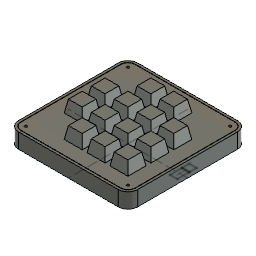
OpenMicro (Autodesk Fusion 360 design; units mm, degrees)
Autodesk Fusion 360 part; units mm, degrees
note: some values were not read from the file. Chosen so that the rebuilt part matches the saved one: which bodies a step acts on.
sketch "Sketch1" plane through (0, 0, 0) normal (0, 1, 0) x (1, 0, 0)
  line L0 (6, 0) -> (89, 0)
  line L1 (95, -6) -> (95, -89)
  line L2 (89, -95) -> (6, -95)
  line L3 (0, -89) -> (0, -6)
  arc A0 (6, 0) -> (0, -6) centre (6, -6) ccw
  arc A1 (95, -6) -> (89, 0) centre (89, -6) ccw
  arc A2 (89, -95) -> (95, -89) centre (89, -89) ccw
  arc A3 (0, -89) -> (6, -95) centre (6, -89) ccw
  line L4 (47.5, 0) -> (47.5, -95) construction
  line L5 (0, -47.5) -> (95, -47.5) construction
  circle A4 centre (5, -5) radius 1
  circle A5 centre (90, -5) radius 1
  circle A6 centre (90, -90) radius 1
  circle A7 centre (5, -90) radius 1
  point P0 (95, 0)
  point P1 (95, -95)
  dimension "d1" = 95
  dimension "d2" = 95
  dimension "d3" = 6
  dimension "d4" = 2
  dimension "d5" = 42.5
  dimension "d6" = 42.5
  constraint horizontal L0
  constraint vertical L1
  constraint horizontal L2
  constraint vertical L3
  constraint coincident origin L0
  constraint coincident origin L3
  constraint tangent L0 A0
  constraint tangent L3 A0
  constraint coincident P0 L0
  constraint coincident P0 L1
  constraint tangent L0 A1
  constraint tangent L1 A1
  constraint equal A0 A1
  constraint coincident P1 L1
  constraint coincident P1 L2
  constraint tangent L1 A2
  constraint tangent L2 A2
  constraint equal A0 A2
  constraint tangent L2 A3
  constraint tangent L3 A3
  constraint equal A0 A3
  constraint midpoint L0 L4.start
  constraint midpoint L2 L4.end
  constraint midpoint L3 L5.start
  constraint midpoint L1 L5.end
  constraint symmetric L4 A4 A5
  constraint symmetric L5 A5 A6
  constraint symmetric L4 A6 A7
  measures "d1" distance of origin P0
  measures "d2" distance of P0 P1
  measures "d3" radius of A0
  measures "d4" diameter of A4
  measures "d5" distance of L4 A4.centre
  measures "d6" distance of L5 A4.centre
extrude "Extrude1" add sketch "Sketch1" along normal blind 1.6 makes body 1
sketch "Sketch2" plane through (0, 1.6, 0) normal (0, 1, 0) x (-1, 0, 0)
  circle A0 centre (-5, 5) radius 1
  circle A1 centre (-5, 90) radius 1
  circle A2 centre (-90, 90) radius 1
  circle A3 centre (-90, 5) radius 1
  arc A4 (-6, 0) -> (0, 6) centre (-6, 6) ccw
  line L0 (0, 6) -> (0, 89)
  arc A5 (0, 89) -> (-6, 95) centre (-6, 89) ccw
  line L1 (-6, 95) -> (-89, 95)
  arc A6 (-89, 95) -> (-95, 89) centre (-89, 89) ccw
  line L2 (-95, 89) -> (-95, 6)
  arc A7 (-95, 6) -> (-89, 0) centre (-89, 6) ccw
  line L3 (-89, 0) -> (-6, 0)
  line L4 (-30.475, 11.425) -> (-45.475, 11.425)
  line L5 (-45.475, 11.425) -> (-45.475, 26.425)
  line L6 (-45.475, 26.425) -> (-30.475, 26.425)
  line L7 (-30.475, 26.425) -> (-30.475, 11.425)
  line L8 (-49.525, 11.425) -> (-64.525, 11.425)
  line L9 (-64.525, 11.425) -> (-64.525, 26.425)
  line L10 (-64.525, 26.425) -> (-49.525, 26.425)
  line L11 (-49.525, 26.425) -> (-49.525, 11.425)
  line L12 (-11.425, 30.475) -> (-26.425, 30.475)
  line L13 (-26.425, 30.475) -> (-26.425, 45.475)
  line L14 (-26.425, 45.475) -> (-11.425, 45.475)
  line L15 (-11.425, 45.475) -> (-11.425, 30.475)
  line L16 (-30.475, 30.475) -> (-45.475, 30.475)
  line L17 (-45.475, 30.475) -> (-45.475, 45.475)
  line L18 (-45.475, 45.475) -> (-30.475, 45.475)
  line L19 (-30.475, 45.475) -> (-30.475, 30.475)
  line L20 (-49.525, 30.475) -> (-64.525, 30.475)
  line L21 (-64.525, 30.475) -> (-64.525, 45.475)
  line L22 (-64.525, 45.475) -> (-49.525, 45.475)
  line L23 (-49.525, 45.475) -> (-49.525, 30.475)
  line L24 (-68.575, 30.475) -> (-83.575, 30.475)
  line L25 (-83.575, 30.475) -> (-83.575, 45.475)
  line L26 (-83.575, 45.475) -> (-68.575, 45.475)
  line L27 (-68.575, 45.475) -> (-68.575, 30.475)
  line L28 (-11.425, 49.525) -> (-26.425, 49.525)
  line L29 (-26.425, 49.525) -> (-26.425, 64.525)
  line L30 (-26.425, 64.525) -> (-11.425, 64.525)
  line L31 (-11.425, 64.525) -> (-11.425, 49.525)
  line L32 (-30.475, 49.525) -> (-45.475, 49.525)
  line L33 (-45.475, 49.525) -> (-45.475, 64.525)
  line L34 (-45.475, 64.525) -> (-30.475, 64.525)
  line L35 (-30.475, 64.525) -> (-30.475, 49.525)
  line L36 (-49.525, 49.525) -> (-64.525, 49.525)
  line L37 (-64.525, 49.525) -> (-64.525, 64.525)
  line L38 (-64.525, 64.525) -> (-49.525, 64.525)
  line L39 (-49.525, 64.525) -> (-49.525, 49.525)
  line L40 (-68.575, 49.525) -> (-83.575, 49.525)
  line L41 (-83.575, 49.525) -> (-83.575, 64.525)
  line L42 (-83.575, 64.525) -> (-68.575, 64.525)
  line L43 (-68.575, 64.525) -> (-68.575, 49.525)
  line L44 (-30.475, 68.575) -> (-45.475, 68.575)
  line L45 (-45.475, 68.575) -> (-45.475, 83.575)
  line L46 (-45.475, 83.575) -> (-30.475, 83.575)
  line L47 (-30.475, 83.575) -> (-30.475, 68.575)
  line L48 (-49.525, 68.575) -> (-64.525, 68.575)
  line L49 (-64.525, 68.575) -> (-64.525, 83.575)
  line L50 (-64.525, 83.575) -> (-49.525, 83.575)
  line L51 (-49.525, 83.575) -> (-49.525, 68.575)
  line L52 (-68.575, 68.575) -> (-83.575, 68.575)
  line L53 (-83.575, 68.575) -> (-83.575, 83.575)
  line L54 (-83.575, 83.575) -> (-68.575, 83.575)
  line L55 (-68.575, 83.575) -> (-68.575, 68.575)
  line L56 (-47.5, 0) -> (-47.5, 95) construction
  line L57 (0, 47.5) -> (-95, 47.5) construction
  line L58 (-37.975, 11.425) -> (-37.975, 26.425) construction
  line L59 (-57.025, 11.425) -> (-57.025, 26.425) construction
  line L60 (-30.475, 18.925) -> (-45.475, 18.925) construction
  line L61 (-18.925, 30.475) -> (-18.925, 45.475) construction
  line L62 (-11.425, 37.975) -> (-26.425, 37.975) construction
  line L63 (-11.425, 57.025) -> (-26.425, 57.025) construction
  line L64 (-76.075, 30.475) -> (-76.075, 45.475) construction
  line L65 (-30.475, 76.075) -> (-45.475, 76.075) construction
  dimension "d9" = 15
  dimension "d10" = 9.525
  dimension "d11" = 28.575
  dimension "d12" = 9.525
  dimension "d13" = 28.575
  dimension "d14" = 9.525
  dimension "d15" = 28.575
  dimension "d16" = 9.525
  dimension "d17" = 28.575
  constraint horizontal L4
  constraint vertical L5
  constraint horizontal L6
  constraint vertical L7
  constraint horizontal L8
  constraint vertical L9
  constraint horizontal L10
  constraint vertical L11
  constraint horizontal L12
  constraint vertical L13
  constraint horizontal L14
  constraint vertical L15
  constraint horizontal L16
  constraint vertical L17
  constraint horizontal L18
  constraint vertical L19
  constraint horizontal L20
  constraint vertical L21
  constraint horizontal L22
  constraint vertical L23
  constraint horizontal L24
  constraint vertical L25
  constraint horizontal L26
  constraint vertical L27
  constraint horizontal L28
  constraint vertical L29
  constraint horizontal L30
  constraint vertical L31
  constraint horizontal L32
  constraint vertical L33
  constraint horizontal L34
  constraint vertical L35
  constraint horizontal L36
  constraint vertical L37
  constraint horizontal L38
  constraint vertical L39
  constraint horizontal L40
  constraint vertical L41
  constraint horizontal L42
  constraint vertical L43
  constraint horizontal L44
  constraint vertical L45
  constraint horizontal L46
  constraint vertical L47
  constraint horizontal L48
  constraint vertical L49
  constraint horizontal L50
  constraint vertical L51
  constraint horizontal L52
  constraint vertical L53
  constraint horizontal L54
  constraint vertical L55
  constraint equal L4 L7
  constraint equal L4 L8
  constraint equal L8 L11
  constraint equal L8 L24
  constraint equal L11 L27
  constraint equal L8 L20
  constraint equal L11 L23
  constraint equal L16 L20
  constraint equal L19 L23
  constraint equal L12 L16
  constraint equal L15 L19
  constraint equal L12 L28
  constraint equal L15 L31
  constraint equal L28 L32
  constraint equal L28 L35
  constraint equal L32 L36
  constraint equal L35 L39
  constraint equal L36 L40
  constraint equal L39 L43
  constraint equal L40 L52
  constraint equal L43 L55
  constraint equal L48 L52
  constraint equal L51 L55
  constraint equal L44 L48
  constraint equal L47 L51
  constraint collinear L15 L31
  constraint collinear L7 L19
  constraint collinear L19 L35
  constraint collinear L35 L47
  constraint collinear L11 L23
  constraint collinear L23 L39
  constraint collinear L39 L51
  constraint collinear L27 L43
  constraint collinear L43 L55
  constraint collinear L4 L8
  constraint collinear L12 L16
  constraint collinear L16 L20
  constraint collinear L20 L24
  constraint collinear L28 L32
  constraint collinear L32 L36
  constraint collinear L36 L40
  constraint collinear L44 L48
  constraint collinear L48 L52
  constraint midpoint L3 L56.start
  constraint midpoint L1 L56.end
  constraint midpoint L0 L57.start
  constraint midpoint L2 L57.end
  constraint midpoint L4 L58.start
  constraint midpoint L6 L58.end
  constraint midpoint L8 L59.start
  constraint midpoint L10 L59.end
  constraint midpoint L7 L60.start
  constraint midpoint L5 L60.end
  constraint midpoint L12 L61.start
  constraint midpoint L14 L61.end
  constraint midpoint L15 L62.start
  constraint midpoint L13 L62.end
  constraint midpoint L31 L63.start
  constraint midpoint L29 L63.end
  constraint midpoint L24 L64.start
  constraint midpoint L26 L64.end
  constraint midpoint L47 L65.start
  constraint midpoint L45 L65.end
  measures "d9" distance of L4.start L4.end
  measures "d10" distance of L56 L58
  measures "d11" distance of L57 L60
  measures "d12" distance of L56 L59
  measures "d13" distance of L56 L61
  measures "d14" distance of L57 L62
  measures "d15" distance of L56 L64
  measures "d16" distance of L57 L63
  measures "d17" distance of L57 L65
extrude "Extrude2" add sketch "Sketch2" along normal blind 10 draft -10 contours L4 L5 L6 L7 | L8 L9 L10 L11 | L12 L13 L14 L15 | L16 L17 L18 L19 | L20 L21 L22 L23 | L24 L25 L26 L27 | L28 L29 L30 L31 | L32 L33 L34 L35 | L36 L37 L38 L39 | L40 L41 L42 L43 | L44 L45 L46 L47 | L48 L49 L50 L51 | L52 L53 L54 L55 bodies 1
sketch "Sketch3" plane through (0, 0, 0) normal (0, -1, 0) x (1, 0, 0)
  circle A0 centre (5, 5) radius 1
  circle A1 centre (5, 90) radius 1
  circle A2 centre (90, 90) radius 1
  circle A3 centre (90, 5) radius 1
  arc A4 (0, 6) -> (6, 0) centre (6, 6) ccw
  line L0 (6, 0) -> (89, 0)
  arc A5 (89, 0) -> (95, 6) centre (89, 6) ccw
  line L1 (95, 6) -> (95, 89)
  arc A6 (95, 89) -> (89, 95) centre (89, 89) ccw
  line L2 (89, 95) -> (6, 95)
  arc A7 (6, 95) -> (0, 89) centre (6, 89) ccw
  line L3 (0, 89) -> (0, 6)
  circle A8 centre (5, 90) radius 1
  circle A9 centre (90, 90) radius 1
  circle A10 centre (90, 5) radius 1
  circle A11 centre (5, 5) radius 1
  circle A12 centre (5, 90) radius 3
  circle A13 centre (90, 90) radius 3
  circle A14 centre (5, 5) radius 3
  circle A15 centre (90, 5) radius 3
  circle A16 centre (5, 5) radius 1.5
  circle A17 centre (90, 5) radius 1.5
  circle A18 centre (90, 90) radius 1.5
  circle A19 centre (5, 90) radius 1.5
  dimension "d20" = 6
  dimension "d21" = 6
  dimension "d22" = 6
  dimension "d23" = 6
  dimension "d44" = 3
  dimension "d45" = 3
  dimension "d46" = 3
  dimension "d47" = 3
  constraint concentric A8 A12
  constraint concentric A9 A13
  constraint concentric A11 A14
  constraint concentric A10 A15
  constraint concentric A14 A16
  constraint concentric A15 A17
  constraint concentric A13 A18
  constraint concentric A12 A19
  measures "d20" diameter of A12
  measures "d21" diameter of A13
  measures "d22" diameter of A14
  measures "d23" diameter of A15
  measures "d44" diameter of A16
  measures "d45" diameter of A17
  measures "d46" diameter of A18
  measures "d47" diameter of A19
extrude "Extrude3" add sketch "Sketch3" along normal blind 5 separate body contours A12 | A13 | A14 | A15 makes body 2 at (88.0149, -3.3333, 87.7507) makes body 3 at (92.9963, -3.3333, 4.8505) makes body 4 at (7.8191, -3.3333, 88.9739) makes body 5 at (7.9963, -3.3333, 4.8505)
sketch "Sketch4" plane through (0, -5, 0) normal (0, -1, 0) x (1, 0, 0)
  circle A0 centre (5, 90) radius 3
  line L0 (89, 95) -> (6, 95)
  arc A1 (6, 95) -> (0, 89) centre (6, 89) ccw
  line L1 (0, 89) -> (0, 6)
  arc A2 (0, 6) -> (6, 0) centre (6, 6) ccw
  line L2 (6, 0) -> (89, 0)
  arc A3 (89, 0) -> (95, 6) centre (89, 6) ccw
  line L3 (95, 6) -> (95, 89)
  arc A4 (95, 89) -> (89, 95) centre (89, 89) ccw
  line L4 (-2.2, 89) -> (-2.2, 6)
  arc A5 (-2.2, 6) -> (6, -2.2) centre (6, 6) ccw
  line L5 (6, -2.2) -> (89, -2.2)
  arc A6 (89, -2.2) -> (97.2, 6) centre (89, 6) ccw
  line L6 (97.2, 6) -> (97.2, 89)
  arc A7 (97.2, 89) -> (89, 97.2) centre (89, 89) ccw
  line L7 (89, 97.2) -> (6, 97.2)
  arc A8 (6, 97.2) -> (-2.2, 89) centre (6, 89) ccw
  circle A9 centre (5, 90) radius 1.5
  dimension "d28" = 2.2
extrude "Extrude4" add sketch "Sketch4" along normal blind 6 contours A0 | L0 A1 L1 A2 L2 A3 L3 A4 | L4 A5 L5 A6 L6 A7 L7 A8 | A9 bodies 2 3 4 5
sketch "Sketch5" plane through (0, -5, 0) normal (0, 1, 0) x (-1, 0, 0)
  arc A0 (2.2, 89) -> (-6, 97.2) centre (-6, 89) ccw
  line L0 (-6, 97.2) -> (-89, 97.2)
  arc A1 (-89, 97.2) -> (-97.2, 89) centre (-89, 89) ccw
  line L1 (-97.2, 89) -> (-97.2, 6)
  arc A2 (-97.2, 6) -> (-89, -2.2) centre (-89, 6) ccw
  line L2 (-89, -2.2) -> (-6, -2.2)
  arc A3 (-6, -2.2) -> (2.2, 6) centre (-6, 6) ccw
  line L3 (2.2, 6) -> (2.2, 89)
  circle A4 centre (-5, 5) radius 3
  circle A5 centre (-90, 5) radius 3
  circle A6 centre (-90, 90) radius 3
  circle A7 centre (-5, 90) radius 3
  line L4 (-95.2, 89) -> (-95.2, 6)
  arc A8 (-95.2, 6) -> (-89, -0.2) centre (-89, 6) ccw
  line L5 (-89, -0.2) -> (-6, -0.2)
  arc A9 (-6, -0.2) -> (0.2, 6) centre (-6, 6) ccw
  line L6 (0.2, 6) -> (0.2, 89)
  arc A10 (0.2, 89) -> (-6, 95.2) centre (-6, 89) ccw
  line L7 (-6, 95.2) -> (-89, 95.2)
  arc A11 (-89, 95.2) -> (-95.2, 89) centre (-89, 89) ccw
  dimension "d29" = -2
extrude "Extrude5" add sketch "Sketch5" along normal blind 6.6 contours A0 L0 A1 L1 A2 L2 A3 L3 bodies 2
sketch "Sketch6" plane through (0, 0, 0) normal (-1, 0, 0) x (0, 0, 1)
  line L0 (6, 0) -> (89, 0)
  line L1 (89, 0) -> (89, 1.6)
  line L2 (89, 1.6) -> (6, 1.6)
  line L3 (6, 1.6) -> (6, 0)
  line L4 (44.46, -0.1) -> (50.54, -0.1)
  line L5 (51.82, -1.38) -> (51.82, -2.08)
  line L6 (50.54, -3.36) -> (44.46, -3.36)
  line L7 (43.18, -2.08) -> (43.18, -1.38)
  line L8 (47.5, 1.6) -> (47.5, 0) construction
  arc A0 (44.46, -0.1) -> (43.18, -1.38) centre (44.46, -1.38) ccw
  arc A1 (51.82, -1.38) -> (50.54, -0.1) centre (50.54, -1.38) ccw
  arc A2 (50.54, -3.36) -> (51.82, -2.08) centre (50.54, -2.08) ccw
  arc A3 (43.18, -2.08) -> (44.46, -3.36) centre (44.46, -2.08) ccw
  point P0 (43.18, -0.1)
  point P1 (51.82, -0.1)
  point P2 (51.82, -3.36)
  dimension "d32" = 8.64
  dimension "d33" = 3.26
  dimension "d35" = 1.28
  dimension "d43" = 0.1
  constraint horizontal L4
  constraint vertical L5
  constraint horizontal L6
  constraint vertical L7
  constraint midpoint L2 L8.start
  constraint midpoint L0 L8.end
  constraint symmetric L5 L7 L8
  constraint coincident P0 L4
  constraint coincident P0 L7
  constraint tangent L4 A0
  constraint tangent L7 A0
  constraint coincident P1 L4
  constraint coincident P1 L5
  constraint tangent L4 A1
  constraint tangent L5 A1
  constraint equal A0 A1
  constraint coincident P2 L5
  constraint coincident P2 L6
  constraint tangent L5 A2
  constraint tangent L6 A2
  constraint equal A0 A2
  constraint tangent L6 A3
  constraint tangent L7 A3
  constraint equal A0 A3
  measures "d32" distance of P0 P1
  measures "d33" distance of P1 P2
  measures "d35" radius of A0
  measures "d43" distance of L0 L4
extrude "Extrude6" add sketch "Sketch6" along normal blind 2 and the other way blind 5.32 separate body contours L4 L5 L6 L7 A0 A1 A2 A3 makes body 6
sketch "Sketch7" plane through (-2.2, 0, 0) normal (-1, 0, 0) x (0, 0, 1)
  line L0 (6, 1.6) -> (6, -11)
  line L1 (6, -11) -> (89, -11)
  line L2 (89, -11) -> (89, 1.6)
  line L3 (89, 1.6) -> (6, 1.6)
  line L4 (50.54, -0.1) -> (44.46, -0.1)
  arc A0 (51.82, -1.38) -> (50.54, -0.1) centre (50.54, -1.38) ccw
  line L5 (51.82, -2.08) -> (51.82, -1.38)
  arc A1 (50.54, -3.36) -> (51.82, -2.08) centre (50.54, -2.08) ccw
  line L6 (44.46, -3.36) -> (50.54, -3.36)
  arc A2 (43.18, -2.08) -> (44.46, -3.36) centre (44.46, -2.08) ccw
  line L7 (43.18, -1.38) -> (43.18, -2.08)
  arc A3 (44.46, -0.1) -> (43.18, -1.38) centre (44.46, -1.38) ccw
  line L8 (42.68, -1.38) -> (42.68, -2.08)
  arc A4 (42.68, -2.08) -> (44.46, -3.86) centre (44.46, -2.08) ccw
  line L9 (44.46, -3.86) -> (50.54, -3.86)
  arc A5 (50.54, -3.86) -> (52.32, -2.08) centre (50.54, -2.08) ccw
  line L10 (52.32, -2.08) -> (52.32, -1.38)
  arc A6 (52.32, -1.38) -> (50.54, 0.4) centre (50.54, -1.38) ccw
  line L11 (50.54, 0.4) -> (44.46, 0.4)
  arc A7 (44.46, 0.4) -> (42.68, -1.38) centre (44.46, -1.38) ccw
  dimension "d40" = 0.5
extrude "Extrude7" cut sketch "Sketch7" against normal up to surface (2 mm away) contours L4 A0 L5 A1 L6 A2 L7 A3 | L8 A4 L9 A5 L10 A6 L11 A7 bodies 2
sketch "Sketch8" plane through (0, -11, 0) normal (0, -1, 0) x (1, 0, 0)
  arc A0 (6, 97.2) -> (-2.2, 89) centre (6, 89) ccw
  line L0 (-2.2, 89) -> (-2.2, 6)
  arc A1 (-2.2, 6) -> (6, -2.2) centre (6, 6) ccw
  line L1 (6, -2.2) -> (89, -2.2)
  arc A2 (89, -2.2) -> (97.2, 6) centre (89, 6) ccw
  line L2 (97.2, 6) -> (97.2, 89)
  arc A3 (97.2, 89) -> (89, 97.2) centre (89, 89) ccw
  line L3 (89, 97.2) -> (6, 97.2)
  line L4 (93.5, 42.5) -> (87.5, 42.5)
  line L5 (87.5, 42.5) -> (87.5, 52.5)
  line L6 (87.5, 52.5) -> (93.5, 52.5)
  line L7 (93.5, 52.5) -> (93.5, 42.5)
  line L8 (97.2, 47.5) -> (-2.2, 47.5) construction
  line L9 (90.5, 42.5) -> (90.5, 52.5) construction
  line L10 (47.5, -2.2) -> (47.5, 97.2) construction
  line L11 (93.5, 42.5) -> (87.5, 42.5)
  line L12 (87.5, 42.5) -> (87.5, 36.5)
  line L13 (87.5, 36.5) -> (93.5, 36.5)
  line L14 (93.5, 36.5) -> (93.5, 42.5)
  dimension "d49" = 43
  dimension "d50" = 6
  dimension "d51" = 10
  dimension "d54" = 6
  constraint horizontal L4
  constraint vertical L5
  constraint horizontal L6
  constraint vertical L7
  constraint midpoint L2 L8.start
  constraint midpoint L0 L8.end
  constraint symmetric L4 L6 L8
  constraint midpoint L4 L9.start
  constraint midpoint L6 L9.end
  constraint midpoint L1 L10.start
  constraint midpoint L3 L10.end
  constraint horizontal L11
  constraint vertical L12
  constraint horizontal L13
  constraint vertical L14
  constraint collinear L5 L12
  measures "d49" distance of L9 L10
  measures "d50" distance of L4.start L4.end
  measures "d51" distance of L4.end L5.end
  measures "d54" distance of L4.end L12.end
extrude "Extrude8" [suppressed]
